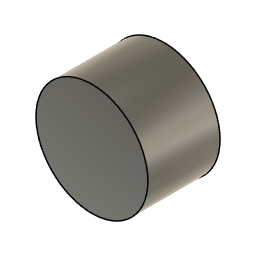
umi_pen_end_effector (Autodesk Fusion 360 archive; units mm, degrees)
design "gripper_iPhoneMax_v1 - bottom_plate"
Autodesk Fusion 360 part; units mm, degrees
sketch "Sketch1" plane through (0, 0, 0) normal (0, 0, 1) x (1, 0, 0)
  line L0 (94.5847, -33.3218, -10) -> (6.5095, -33.3218, -10)
  line L1 (6.5095, -33.3218, -10) -> (6.5095, 73.9441, -10)
  line L2 (6.5095, 73.9441, -10) -> (94.5847, 73.9441, -10)
  line L3 (94.5847, 73.9441, -10) -> (94.5847, -33.3218, -10)
sketch "Sketch2" plane through (0, 0, 0) normal (0, 1, 0) x (1, 0, 0)
  circle A0 centre (-0.0361, -7.2532) radius 6.2056
extrude "Extrude2" add sketch "Sketch2" along normal blind 11
hole "Hole1" at (-1.2862, 11, 9.8296) direction (0, -1, 0) diameter 19 depth 3 tip angle 180
hole "Hole2" at (-0.0361, 8, 7.2532) direction (0, -1, 0) diameter 11 depth 3 tip angle 180
